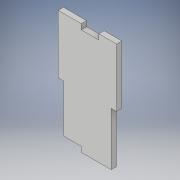
# Autodesk Inventor part: fromt_right
Saved by Autodesk Inventor 2017.2 (Build 212233000, 233)
## iProperties
Created: 2017-06-02
Part Number: fromt_right
Material: Generic
Document SubType Name: Modeling
Designer: SandeepSH
Density: 1 g/cm^3
Appearance: Default
Author: SandeepSH
Autodesk Inventor part; units mm, degrees
ref_plane "YZ Plane" through (0, 0, 0) normal (1, 0, 0) x (0, 1, 0)
ref_plane "XZ Plane" through (0, 0, 0) normal (0, 1, 0) x (-1, 0, 0)
ref_plane "XY Plane" through (0, 0, 0) normal (0, 0, 1) x (1, 0, 0)
sketch "Sketch1" plane through (0, 0, 0) normal (0, 0, 1) x (1, 0, 0)
  line L0 (-16.5, -31.5) -> (16.5, -31.5)
  line L1 (16.5, -31.5) -> (16.5, 31.5)
  line L2 (16.5, 31.5) -> (-16.5, 31.5)
  line L3 (-16.5, 31.5) -> (-16.5, -31.5)
  line L4 (-16.5, -31.5) -> (16.5, 31.5) construction
  line L5 (16.5, -31.5) -> (-16.5, 31.5) construction
  point P0 (0, 0)
  dimension "d0" = 33
  dimension "d1" = 63
  constraints: 12 end point, 2 midpoint, 2 parallel, 1 horizontal, 1 perpendicular
  measures "d0" distance of L2.end L1.end
  measures "d1" distance of L1.end L0.end
extrude "Extrusion1" add sketch "Sketch1" along normal blind 3
sketch "Sketch2" plane through (0, 0, 3) normal (0, 0, 1) x (1, 0, 0)
  line L0 (-16.5, 31.5) -> (-16.5, -31.5) projected
  line L1 (-16.5, -31.5) -> (-13.5, -31.5)
  line L2 (-13.5, -31.5) -> (-13.5, -1.5)
  line L3 (-13.5, -1.5) -> (-16.5, -1.5)
  line L4 (-16.5, -1.5) -> (-16.5, -31.5)
  line L5 (-16.5, -31.5) -> (16.5, -31.5) projected
  line L6 (16.5, -31.5) -> (13.5, -31.5)
  line L7 (13.5, -31.5) -> (13.5, -1.5)
  line L8 (13.5, -1.5) -> (16.5, -1.5)
  line L9 (16.5, -1.5) -> (16.5, -31.5)
  line L10 (-13.5, -31.5) -> (-3.5, -31.5)
  line L11 (-3.5, -31.5) -> (-3.5, -28.5)
  line L12 (-3.5, -28.5) -> (-13.5, -28.5)
  line L13 (-13.5, -28.5) -> (-13.5, -31.5)
  line L14 (-3.5, 31.5) -> (6.5, 31.5)
  line L15 (6.5, 31.5) -> (6.5, 28.5)
  line L16 (6.5, 28.5) -> (-3.5, 28.5)
  line L17 (-3.5, 28.5) -> (-3.5, 31.5)
  line L18 (16.5, -31.5) -> (16.5, 31.5) projected
  point P0 (0, 0)
  dimension "d4" = 3
  dimension "d5" = 30
  dimension "d6" = 3
  dimension "d7" = 30
  dimension "d8" = 3
  dimension "d9" = 17
  dimension "d10" = 10
  dimension "d11" = 3
  dimension "d12" = 10
  constraints: 32 end point, 8 parallel, 4 horizontal, 4 perpendicular
  measures "d4" distance of L3.end L2.end
  measures "d5" distance of L2.end L1.end
  measures "d6" distance of L7.end L8.end
  measures "d7" distance of L6.end L7.end
  measures "d8" distance of L11.end L10.end
  measures "d9" distance between parallel lines of L7 L11
  measures "d10" distance of L15.end L16.end
  measures "d11" distance of L14.end L15.end
  measures "d12" distance between parallel lines of L18 L15
extrude "Extrusion2" cut sketch "Sketch2" against normal through all
body "Solid1"
